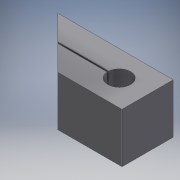
# Autodesk Inventor part: AXTTS
Saved by Autodesk Inventor 2016 (Build 200138000, 138)
## iProperties
Created: 2017-07-16
Part Number: AXTTS
Material: PC/ABS Plastic
Document SubType Name: Modeling
Designer: ludwi
Density: 0.357273 g/cm^3
Appearance: Smooth - White
Author: ludwi
Autodesk Inventor part; units mm, degrees
ref_plane "YZ Plane" through (0, 0, 0) normal (1, 0, 0) x (0, 1, 0)
ref_plane "XZ Plane" through (0, 0, 0) normal (0, 1, 0) x (-1, 0, 0)
ref_plane "XY Plane" through (0, 0, 0) normal (0, 0, 1) x (1, 0, 0)
sketch "Sketch1" plane through (0, 0, 0) normal (0, 0, 1) x (1, 0, 0)
  line L0 (0, 2) -> (100, 2) construction
  line L1 (0, 2) -> (0, 18) construction
  line L2 (12, 18) -> (0, 18) construction
  arc A0 (12, 18) -> (28, 18) centre (20, 18) ccw construction
  line L3 (38, 18) -> (28, 18) construction
  arc A1 (38, 18) -> (62, 18) centre (50, 18) ccw construction
  line L4 (72, 18) -> (62, 18) construction
  arc A2 (72, 18) -> (88, 18) centre (80, 18) ccw construction
  line L5 (100, 18) -> (88, 18) construction
  line L6 (100, 2) -> (100, 18) construction
  line L7 (100, 34) -> (0, 34) construction
  line L8 (100, 34) -> (100, 18) construction
  line L9 (88, 18) -> (100, 18) construction
  arc A3 (88, 18) -> (72, 18) centre (80, 18) ccw construction
  line L10 (62, 18) -> (72, 18) construction
  arc A4 (62, 18) -> (38, 18) centre (50, 18) ccw construction
  line L11 (28, 18) -> (38, 18) construction
  arc A5 (28, 18) -> (12, 18) centre (20, 18) ccw construction
  line L12 (0, 18) -> (12, 18) construction
  line L13 (0, 34) -> (0, 18) construction
  line L14 (100, 2) -> (100, 0) construction
  line L15 (100, 0) -> (0, 0) construction
  line L16 (0, 0) -> (0, 2) construction
  line L17 (0, 2) -> (100, 2) construction
  line L18 (0, 34) -> (0, 36) construction
  line L19 (0, 36) -> (100, 36) construction
  line L20 (100, 36) -> (100, 34) construction
  line L21 (100, 34) -> (0, 34) construction
  line L22 (100, 36) -> (100, 0)
  line L23 (100, 0) -> (55, 0)
  line L24 (19, 36) -> (100, 36)
  circle A6 centre (80, 18) radius 8
  line L25 (72.0156, 18.5) -> (36.5, 18.5)
  line L26 (37.5, 17.5) -> (72.0156, 17.5)
  line L27 (55, 0) -> (37.5, 17.5)
  line L28 (36.5, 18.5) -> (19, 36)
  line L29 (55.9956, 18.5) -> (55.9956, 17.5) construction
  line L30 (36.5, 18.5) -> (37.5, 17.5) construction
  point P0 (55.9956, 18)
  dimension "d1" = 45
  dimension "d3" = 1
  dimension "d4" = 45
  constraints: 18 end point, 4 point on line, 3 collinear, 2 parallel, 2 point on circle, 1 centre point, 1 coincident, 1 concentric, 1 horizontal, 1 horizontal alignment, 1 midpoint, 1 perpendicular
  measures "d1" distance of L14.end L23.end
  measures "d3" distance between parallel lines of L25 L26
  measures "d4" angle of L15 L27
extrude "Extrusion1" add sketch "Sketch1" along normal blind 32 contours L22 L23 L27 L26 A6 L25 L28 L24
sketch "Sketch2" plane through (55, 0, 0) normal (0, -1, 0) x (1, 0, 0)
  circle A0 centre (38.5, 25.5) radius 3 projected
  circle A1 centre (38.5, 6.5) radius 3 projected
  circle A2 centre (8.7, 16) radius 3 projected
  point P0 (-55, 0)
extrude "Extrusion2" cut sketch "Sketch2" against normal through all
chamfer "Chamfer1" distance 2 angle 45 4 edges at (77.5, 0, 0) (59.5, 36, 0) (77.5, 0, 32) (59.5, 36, 32)
body "Solid1"
